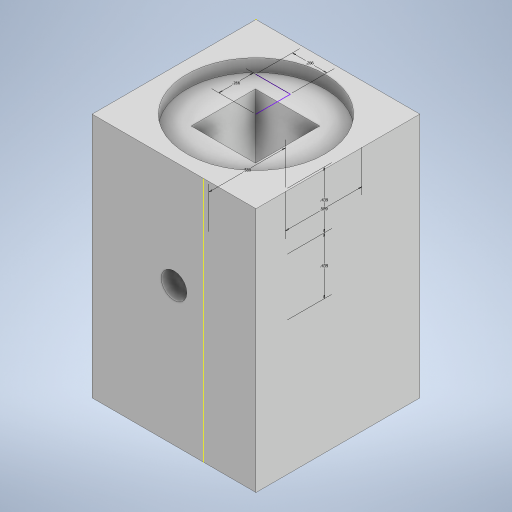
# Autodesk Inventor part: alan_optics_through_hole_chl_turbidity
Saved by Autodesk Inventor 2024 (Build 280153000, 153)
## iProperties
Created: 2024-02-20
Part Number: alan_optics_through_hole_chl_turbidity
Material: Generic
Document SubType Name: Modeling
Designer: jtw4137
Density: 1 g/cm^3
Appearance: Default
Author: jtw4137
Autodesk Inventor part; units mm, degrees
ref_plane "YZ Plane" through (0, 0, 0) normal (1, 0, 0) x (0, 1, 0)
ref_plane "XZ Plane" through (0, 0, 0) normal (0, 1, 0) x (-1, 0, 0)
ref_plane "XY Plane" through (0, 0, 0) normal (0, 0, 1) x (1, 0, 0)
sketch "Sketch3" plane through (0, 0, 0) normal (0, 0, 1) x (1, 0, 0)
  line L0 (0, 0) -> (32, 0)
  line L1 (32, 0) -> (32, 48)
  line L2 (32, 48) -> (0, 48)
  line L3 (0, 48) -> (0, 0)
  dimension "d8" = 32
  dimension "d9" = 48
  constraints: 8 end point, 3 perpendicular, 1 horizontal
  measures "d8" distance of L0.start L0.end
  measures "d9" distance of L0.end L1.end
extrude "Extrusion2" add sketch "Sketch3" along normal blind 32
sketch "Sketch4" plane through (0, 48, 0) normal (0, 1, 0) x (1, 0, 0)
  line L0 (32, -32) -> (0, -32) projected
  line L1 (0, -32) -> (0, -16)
  line L2 (0, 0) -> (0, -32) projected
  line L3 (0, -16) -> (16, -16)
  circle A0 centre (16, -16) radius 13.5
  dimension "d12" = 16
  dimension "d13" = 16
  dimension "d14" = 27
  constraints: 4 end point, 1 centre point, 1 coincident, 1 midpoint, 1 perpendicular
  measures "d12" distance of L0.end L1.end
  measures "d13" distance of L1.end L3.end
  measures "d14" diameter of A0
sketch "Sketch5" plane through (0, 48, 0) normal (0, 1, 0) x (1, 0, 0)
  line L0 (15.9518, -16.0315) -> (15.9518, -9.2765)
  line L1 (15.9518, -9.2765) -> (9.1968, -9.2765)
  point P0 (0, 0)
  dimension "d15" = 6.755
  dimension "d16" = 6.755
  constraints: 4 end point, 1 perpendicular, 1 vertical
  measures "d15" distance of L0.start L0.end
  measures "d16" distance of L0.end L1.end
sketch "Sketch6" plane through (0, 48, 0) normal (0, 1, 0) x (1, 0, 0)
  line L0 (9.1912, -9.2989) -> (9.1912, -21.8489)
  line L1 (9.1912, -21.8489) -> (21.7412, -21.8489)
  line L2 (21.7412, -21.8489) -> (21.7412, -9.2989)
  line L3 (21.7412, -9.2989) -> (9.1912, -9.2989)
  point P0 (0, 0)
  dimension "d17" = 12.55
  dimension "d18" = 12.55
  dimension "d19" = 12.55
  dimension "d20" = 12.55
  constraints: 8 end point, 2 perpendicular, 1 vertical
  measures "d17" distance of L0.start L0.end
  measures "d18" distance of L0.end L1.end
  measures "d19" distance of L1.end L2.end
  measures "d20" distance of L2.end L0.start
extrude "Extrusion4" cut sketch "Sketch6" against normal blind 36
sketch "Sketch7" plane through (0, 0, 32) normal (0, 0, 1) x (1, 0, 0)
  line L0 (32, 48) -> (0, 48) projected
  line L1 (0, 48) -> (16, 48)
  line L2 (16, 48) -> (16, 27)
  circle A0 centre (16, 27) radius 2.5
  point P0 (0, 0)
  dimension "d25" = 16
  dimension "d26" = 21
  dimension "d27" = 5
  constraints: 4 end point, 1 centre point, 1 coincident, 1 midpoint, 1 vertical
  measures "d25" distance of L0.end L1.end
  measures "d26" distance of L1.end L2.end
  measures "d27" diameter of A0
hole "Hole1" at (16, 27, 32) direction (0, 0, -1) diameter 5 end through all
sketch "Sketch9" plane through (0, 0, 0) normal (-1, 0, 0) x (0, 0, 1)
  line L0 (0, 48) -> (16, 48)
  line L1 (21.8489, 48) -> (9.2989, 48) projected
  line L2 (16, 48) -> (16, 27)
  circle A0 centre (16, 27) radius 2.5
  point P0 (0, 0)
  dimension "d37" = 16
  dimension "d38" = 21
  dimension "d39" = 5
  constraints: 4 end point, 1 centre point, 1 coincident, 1 perpendicular, 1 point on line
  measures "d37" distance of L0.start L0.end
  measures "d38" distance of L0.end L2.end
  measures "d39" diameter of A0
hole "Hole2" at (0, 27, 16) direction (1, 0, 0) diameter 5 depth 10 tip angle 118
sketch "Sketch10" plane through (21.7412, 48, 9.2989) normal (-1, 0, 0) x (0, 0, 1)
  circle A0 centre (6.7011, -21) radius 2.5 projected
  line L0 (6.7011, -21) -> (6.7011, -9.86)
  line L1 (6.7011, -9.86) -> (6.7011, -21)
  line L2 (6.7011, -21) -> (6.7011, -9.86)
  line L3 (6.7011, -21) -> (6.7011, -32.14)
  line L4 (12.55, -36) -> (0, -36) projected
  line L5 (6.7011, -32.14) -> (6.7011, -21)
  line L6 (6.7011, -9.86) -> (21.6511, -9.86)
  line L7 (22.7011, -48) -> (22.7011, 0) projected
  line L8 (21.6511, -9.86) -> (6.7011, -9.86)
  line L9 (6.7011, -9.86) -> (-8.2489, -9.86)
  line L10 (21.6511, -9.86) -> (19.0973, -9.86)
  point P0 (-9.2989, -48)
  dimension "d47" = 11.14
  dimension "d48" = 11.14
  dimension "d49" = 14.95
  dimension "d50" = 14.95
  constraints: 18 end point, 4 collinear, 2 perpendicular, 2 point on line, 1 vertical
  measures "d47" distance of L0.start L0.end
  measures "d48" distance of L0.start L3.end
  measures "d49" distance of L0.end L6.end
  measures "d50" distance of L0.end L9.end
sketch "Sketch11" plane through (0, 0, 0) normal (-1, 0, 0) x (0, 0, 1)
  line L0 (16.1419, 38.0227) -> (31.0919, 38.0227)
  line L1 (31.0919, 38.0227) -> (31.0919, 15.7427)
  line L2 (31.0919, 15.7427) -> (1.1919, 15.7427)
  line L3 (1.1919, 15.7427) -> (1.1919, 38.0227)
  line L4 (1.1919, 38.0227) -> (16.1419, 38.0227)
  line L5 (1.1919, 38.0227) -> (6.1919, 38.0227)
  line L6 (6.1919, 38.0227) -> (6.1919, 33.0227)
  circle A0 centre (6.1919, 33.0227) radius 1.7416
  point P0 (0, 0)
  dimension "d51" = 14.95
  dimension "d52" = 22.28
  dimension "d53" = 29.9
  dimension "d54" = 5
  dimension "d55" = 5
  constraints: 14 end point, 5 perpendicular, 2 point on line, 1 centre point, 1 coincident, 1 horizontal
  measures "d51" distance of L0.start L0.end
  measures "d52" distance of L0.end L1.end
  measures "d53" distance of L1.end L2.end
  measures "d54" distance of L3.end L5.end
  measures "d55" distance of L5.end L6.end
hole "Hole3" at (0, 33.0227, 6.1919) direction (1, 0, 0) diameter 3 depth 8 tip angle 118
sketch "Sketch12" plane through (0, 0, 0) normal (-1, 0, 0) x (0, 0, 1)
  point P0 (0, 0)
sketch "Sketch13" plane through (0, 0, 0) normal (-1, 0, 0) x (0, 0, 1)
  line L0 (30.9396, 38.5646) -> (25.9396, 38.5646)
  line L1 (25.9396, 38.5646) -> (25.9396, 33.5646)
  circle A0 centre (25.9396, 33.5646) radius 1.5
  point P0 (0, 0)
  dimension "d63" = 5
  dimension "d64" = 5
  dimension "d65" = 3
  constraints: 4 end point, 1 centre point, 1 coincident, 1 horizontal, 1 perpendicular
  measures "d63" distance of L0.start L0.end
  measures "d64" distance of L0.end L1.end
  measures "d65" diameter of A0
hole "Hole4" at (0, 33.5646, 25.9396) direction (1, 0, 0) diameter 3 depth 8 tip angle 118
sketch "Sketch14" plane through (0, 0, 0) normal (-1, 0, 0) x (0, 0, 1)
  line L0 (15.9777, 27.06) -> (1.0277, 27.06)
  line L1 (1.0277, 27.06) -> (1.0277, 15.92)
  line L2 (1.0277, 15.92) -> (6.0277, 15.92)
  line L3 (6.0277, 15.92) -> (6.0277, 20.92)
  circle A0 centre (6.0277, 20.92) radius 1.5
  point P0 (0, 0)
  dimension "d73" = 14.95
  dimension "d74" = 11.14
  dimension "d75" = 5
  dimension "d76" = 5
  dimension "d77" = 3
  constraints: 8 end point, 3 perpendicular, 1 centre point, 1 coincident, 1 horizontal
  measures "d73" distance of L0.start L0.end
  measures "d74" distance of L0.end L1.end
  measures "d75" distance of L1.end L2.end
  measures "d76" distance of L2.end L3.end
  measures "d77" diameter of A0
hole "Hole5" at (0, 20.92, 6.0277) direction (1, 0, 0) diameter 3 depth 8 tip angle 118
sketch "Sketch15" plane through (0, 0, 0) normal (-1, 0, 0) x (0, 0, 1)
  circle A0 centre (16, 27) radius 2.5 projected
  line L0 (16, 27) -> (30.95, 27)
  line L1 (30.95, 27) -> (30.95, 15.86)
  line L2 (30.95, 15.86) -> (25.95, 15.86)
  line L3 (25.95, 15.86) -> (25.95, 20.86)
  circle A1 centre (25.95, 20.86) radius 1.5
  point P0 (0, 0)
  dimension "d85" = 14.95
  dimension "d86" = 11.14
  dimension "d87" = 5
  dimension "d88" = 5
  dimension "d89" = 3
  constraints: 8 end point, 3 perpendicular, 1 centre point, 1 coincident, 1 horizontal
  measures "d85" distance of L0.start L0.end
  measures "d86" distance of L0.end L1.end
  measures "d87" distance of L1.end L2.end
  measures "d88" distance of L2.end L3.end
  measures "d89" diameter of A1
hole "Hole6" at (0, 20.86, 25.95) direction (1, 0, 0) diameter 3 depth 8 tip angle 118
sketch "Sketch16" plane through (0, 0, 0) normal (-1, 0, 0) x (0, 0, 1)
  line L0 (0, 48) -> (0, 0) projected
  line L1 (0.7991, 31.1876) -> (12.4138, 31.1876)
  line L2 (9.2989, 48) -> (9.2989, 12) projected
  line L3 (12.4138, 31.1876) -> (12.4138, 22.9537)
  line L4 (12.4138, 22.9537) -> (0.7991, 22.9537)
  line L5 (0.7991, 22.9537) -> (0.7991, 31.1876)
  constraints: 8 end point, 4 perpendicular
extrude "Extrusion5" cut sketch "Sketch16" against normal blind 1.35
sketch "Sketch17" plane through (0, 0, 0) normal (-1, 0, 0) x (0, 0, 1)
  line L0 (19.8801, 31.1662) -> (30.9916, 31.1662)
  line L1 (30.9916, 31.1662) -> (30.9916, 23.0241)
  line L2 (30.9916, 23.0241) -> (19.8801, 23.0241)
  line L3 (19.8801, 23.0241) -> (19.8801, 31.1662)
  point P0 (0, 0)
  constraints: 8 end point, 3 perpendicular, 1 horizontal
extrude "Extrusion6" cut sketch "Sketch17" against normal blind 1.35
extrude "Extrusion7" cut sketch "Sketch4" against normal blind 2.5
body "Solid2"
